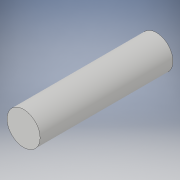
# Autodesk Inventor part: Union
Saved by Autodesk Inventor 2019 (Build 230136000, 136)
## iProperties
Created: 2019-07-03
Part Number: Union
Material: Generic
Document SubType Name: Modeling
Designer: Oscar Rojas
Density: 1 g/cm^3
Appearance: Default
Author: Oscar Rojas
Autodesk Inventor part; units mm, degrees
ref_plane "YZ Plane" through (0, 0, 0) normal (1, 0, 0) x (0, 1, 0)
ref_plane "XZ Plane" through (0, 0, 0) normal (0, 1, 0) x (-1, 0, 0)
ref_plane "XY Plane" through (0, 0, 0) normal (0, 0, 1) x (1, 0, 0)
sketch "Sketch1" plane through (0, 0, 0) normal (0, 0, 1) x (1, 0, 0)
  circle A0 centre (0, 0) radius 2
  dimension "d3" = 4
  constraints: 1 centre point
  measures "d3" diameter of A0
extrude "Extrusion1" add sketch "Sketch1" along normal blind 16.08
body "Solid1"
